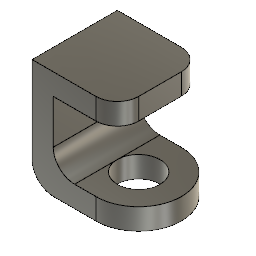
DFAB Exersize 3 v2 (Autodesk Fusion 360 design; units mm, degrees)
Autodesk Fusion 360 part; units mm, degrees
sketch "Sketch3" plane through (0, 0, 0) normal (0, 0, 1) x (1, 0, 0)
  circle A0 centre (0, 0) radius 10
  line L0 (0, 20) -> (-37, 20)
  line L1 (0, -20) -> (-38, -20)
  line L2 (-10, 20) -> (-10, -20)
  line L3 (-20, 20) -> (-20, -20)
  arc A1 (0, -20) -> (0, 20) centre (0, 0) ccw
  line L4 (-30, 20) -> (-30, -20)
  dimension "d7" = 20
  dimension "d8" = 40
  dimension "d10" = 10
  constraint coincident A0.centre A1.centre
  constraint horizontal L0
  constraint parallel L0 L1
  constraint tangent L0 A1
  constraint tangent L1 A1
  constraint coincident L0 L2.start
  constraint coincident L1 L2.end
  constraint perpendicular L1 L2
  constraint tangent A0 L2
  constraint coincident L0 L3.start
  constraint coincident L1 L3.end
  constraint perpendicular L1 L3
  constraint tangent L3 A1
  constraint coincident L0 L4.start
  constraint coincident L1 L4.end
  constraint perpendicular L1 L4
  measures "d7" diameter of A0
  measures "d8" diameter of A1
  measures "d10" distance of L3 L4
extrude "Extrude2" add sketch "Sketch3" along normal blind 10 contours L0 L1 L2 A1 makes body 1
extrude "Extrude3" add sketch "Sketch3" along normal blind 50.6 separate body contours L0 L1 L3 L4 makes body 2
extrude "Extrude4" add sketch "Sketch3" along normal blind 10 contours L0 L1 L2 L3 bodies 1 2
fillet "Fillet1" radius 10 1 edges at (-20, 0, 10) on bodies 1
fillet "Fillet2" radius 10 1 edges at (-30, 0, 0) on bodies 1
sketch "Sketch4" plane through (0, 0, 0) normal (1, 0, 0) x (0, 1, 0)
  line L0 (-20, 50.6, -20) -> (20, 50.6, -20)
  line L1 (20, 50.6, -20) -> (20, 40.6, -20)
  line L2 (20, 40.6, -20) -> (-20, 40.6, -20)
  line L3 (-20, 40.6, -20) -> (-20, 50.6, -20)
  dimension "d19" = 40
  dimension "d20" = 10
extrude "Extrude5" add sketch "Sketch4" along normal blind 30 contours L0 L1 L2 L3 in plane through (-20, 0, 0) normal (1, 0, 0) bodies 1
fillet "Fillet3" radius 10 2 edges at (10, -20, 45.6) (10, 20, 45.6) on bodies 1
